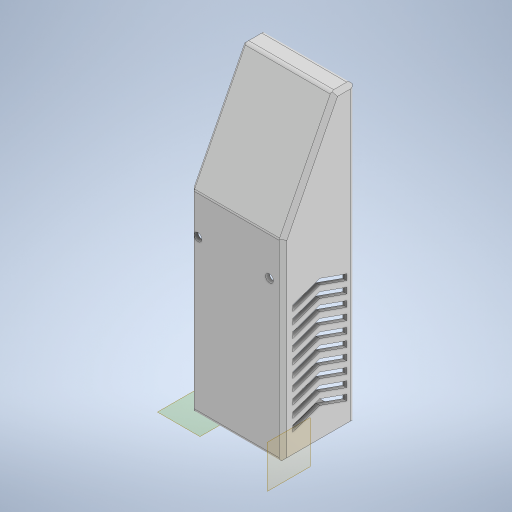
# Autodesk Inventor part: PrawyBłotnik
Saved by Autodesk Inventor 2024 (Build 280153000, 153)
## iProperties
Created: 2025-05-22
Part Number: PrawyBłotnik
Material: Ogólny
Document SubType Name: Modeling
Designer: Victoria
Density: 1 g/cm^3
Appearance: Domyślna
Author: Victoria
Autodesk Inventor part; units mm, degrees
ref_plane "YZ Plane" through (0, 0, 0) normal (1, 0, 0) x (0, 1, 0)
ref_plane "XZ Plane" through (0, 0, 0) normal (0, 1, 0) x (-1, 0, 0)
ref_plane "XY Plane" through (0, 0, 0) normal (0, 0, 1) x (1, 0, 0)
sketch "Szkic1" plane through (0, 0, 0) normal (0, 0, 1) x (1, 0, 0)
  circle A0 centre (16, 0) radius 2
  circle A1 centre (-21, 0) radius 2
  line L0 (-23, 0) -> (-30, 0)
  line L1 (18, 0) -> (23, 0)
  line L2 (23, 0) -> (23, -80)
  line L3 (23, 0) -> (23, 73)
  line L4 (23, 0) -> (96, 0) construction
  line L5 (23, -80) -> (-25, -80)
  line L6 (-25, 73) -> (23, 73)
  line L7 (-25, 73) -> (-25, -80)
  line L8 (-25, 0) -> (-23, 0)
  point P0 (0, 0)
  point P1 (-30, 73)
  point P2 (20.5, 0)
  dimension "d0" = 4
  dimension "d1" = 4
  dimension "d3" = 5
  dimension "d4" = 80
  dimension "d40" = 16
  constraints: 18 end point, 4 horizontal, 2 horizontal alignment, 2 perpendicular, 2 point on line, 1 collinear, 1 midpoint, 1 vertical, 4 other
  measures "d3" distance of L1.start L1.end
  measures "d4" distance of L1.end L2.end
  measures "d40" distance of point (0, 0) point (16, 0)
extrude "Wyciągnięcie proste1" add sketch "Szkic1" along normal blind 2
sketch "Szkic2" plane through (0, 0, 0) normal (0, 0, -1) x (-1, 0, 0)
  line L0 (-23, 73) -> (25, 73) projected
  line L1 (-23, -80) -> (-23, 73) projected
  line L2 (25, -80) -> (-23, -80) projected
  line L3 (25, 73) -> (25, -80) projected
  circle A0 centre (-16, 0) radius 2 projected
  circle A1 centre (21, 0) radius 2 projected
  line L4 (-21, 71) -> (23, 71)
  line L5 (23, 71) -> (23, -78)
  line L6 (23, -78) -> (-21, -78)
  line L7 (-21, -78) -> (-21, 71)
  line L8 (23, 71) -> (25, 71)
  line L9 (23, -78) -> (25, -78)
  line L10 (25, 73) -> (25, -80) projected
  line L11 (23, -68) -> (25, -68)
  line L12 (23, -20) -> (25, -20)
  line L13 (23, 20) -> (25, 20)
  line L14 (23, 10) -> (25, 10)
  point P0 (0, 0)
  dimension "d9" = 2
  constraints: 20 end point, 11 point on line, 5 perpendicular, 3 other
  measures "d9" distance between parallel lines of L1 L7
extrude "Wyciągnięcie proste2" add sketch "Szkic2" along normal blind 35 contours L0 L3 L8 L4 L7 L6 L9 L2 L1 | L3 L13 L5 L8 | L3 L14 L5 L13 | L9 L5 L11 L3
sketch "Szkic3" plane through (23, -80, 2) normal (1, 0, 0) x (0, 0, -1)
  line L0 (37, 153) -> (37, 0) projected
  line L1 (37, 153) -> (27, 153)
  line L2 (0, 0) -> (0, 153) projected
  line L3 (0, 100) -> (27, 153)
  line L4 (0, 100) -> (0, 153)
  line L5 (37, 153) -> (0, 153) projected
  line L6 (27, 153) -> (0, 153)
  point P0 (2, 80)
  dimension "d12" = 10
  dimension "d42" = 20
  constraints: 8 end point, 2 collinear, 1 horizontal, 1 point on line
  measures "d12" distance of L0.start L1.end
  measures "d42" vertical distance of L3.start point (2, 80)
extrude "Wyciągnięcie proste3" cut sketch "Szkic3" against normal up to surface (48 mm away)
sketch "Szkic4" plane through (23, -80, -35) normal (1, 0, 0) x (0, 0, -1)
  line L0 (-37, 100) -> (-10, 153) projected
  line L1 (-37, 100) -> (-35, 100)
  line L2 (-35, 151) -> (-35, 2) projected
  line L3 (0, 153) -> (-10, 153) projected
  line L4 (-10, 153) -> (-8, 153)
  line L5 (-8, 153) -> (-35, 100)
  point P0 (-35, 80)
  point P1 (-35, 103.9259)
  dimension "d15" = 2
  constraints: 6 end point, 2 point on line, 1 horizontal
  measures "d15" distance of L0.end L4.end
extrude "Wyciągnięcie proste4" add sketch "Szkic4" against normal up to surface (48 mm away)
ref_plane "Płaszczyzna konstrukcyjna1" through (23, -77, -1) normal (1, 0, 0) x (0, 0, -1)
sketch "Szkic6" plane through (23, -77, -1) normal (1, 0, 0) x (0, 0, -1)
  line L0 (32, 0) -> (32, 9) projected
  line L1 (32, 9) -> (16, 9)
  line L2 (-1, 9) -> (32, 9) projected
  line L3 (16, 9) -> (16, 95.8634)
  line L4 (16, 9) -> (16, 14)
  line L5 (30, 9) -> (16, 14)
  line L6 (16, 14) -> (2, 9)
  line L7 (30, 9) -> (30, 12)
  line L8 (16, 14) -> (16, 17)
  line L9 (16, 17) -> (30, 12)
  line L10 (2, 9) -> (2, 12)
  line L11 (2, 96.2799) -> (2, 2) projected
  line L12 (2, 12) -> (16, 17)
  line L13 (16, 20) -> (2, 15)
  line L14 (2, 18) -> (16, 23)
  line L15 (2, 15) -> (2, 18)
  line L16 (30, 15) -> (16, 20)
  line L17 (16, 23) -> (30, 18)
  line L18 (30, 15) -> (30, 18)
  line L19 (16, 26) -> (2, 21)
  line L20 (2, 24) -> (16, 29)
  line L21 (2, 21) -> (2, 24)
  line L22 (30, 21) -> (16, 26)
  line L23 (16, 29) -> (30, 24)
  line L24 (30, 21) -> (30, 24)
  line L25 (16, 32) -> (2, 27)
  line L26 (2, 30) -> (16, 35)
  line L27 (2, 27) -> (2, 30)
  line L28 (30, 27) -> (16, 32)
  line L29 (16, 35) -> (30, 30)
  line L30 (30, 27) -> (30, 30)
  line L31 (16, 38) -> (2, 33)
  line L32 (2, 36) -> (16, 41)
  line L33 (2, 33) -> (2, 36)
  line L34 (30, 33) -> (16, 38)
  line L35 (16, 41) -> (30, 36)
  line L36 (30, 33) -> (30, 36)
  line L37 (16, 44) -> (2, 39)
  line L38 (2, 42) -> (16, 47)
  line L39 (2, 39) -> (2, 42)
  line L40 (30, 39) -> (16, 44)
  line L41 (16, 47) -> (30, 42)
  line L42 (30, 39) -> (30, 42)
  line L43 (16, 50) -> (2, 45)
  line L44 (2, 48) -> (16, 53)
  line L45 (2, 45) -> (2, 48)
  line L46 (30, 45) -> (16, 50)
  line L47 (16, 53) -> (30, 48)
  line L48 (30, 45) -> (30, 48)
  line L49 (16, 56) -> (2, 51)
  line L50 (2, 54) -> (16, 59)
  line L51 (2, 51) -> (2, 54)
  line L52 (30, 51) -> (16, 56)
  line L53 (16, 59) -> (30, 54)
  line L54 (30, 51) -> (30, 54)
  line L55 (16, 62) -> (2, 57)
  line L56 (2, 60) -> (16, 65)
  line L57 (2, 57) -> (2, 60)
  line L58 (30, 57) -> (16, 62)
  line L59 (16, 65) -> (30, 60)
  line L60 (30, 57) -> (30, 60)
  line L61 (16, 68) -> (2, 63)
  line L62 (2, 66) -> (16, 71)
  line L63 (2, 63) -> (2, 66)
  line L64 (30, 63) -> (16, 68)
  line L65 (16, 71) -> (30, 66)
  line L66 (30, 63) -> (30, 66)
  point P0 (-1, 77)
  point P1 (0, 9)
  point P2 (16, 71)
  point P3 (2, 63)
  point P4 (16, 65)
  point P5 (2, 57)
  point P6 (16, 59)
  point P7 (2, 54)
  point P8 (2, 51)
  point P9 (16, 53)
  point P10 (2, 48)
  point P11 (2, 45)
  point P12 (2, 39)
  point P13 (2, 33)
  point P14 (2, 27)
  point P15 (16, 29)
  point P16 (2, 21)
  point P17 (16, 23)
  point P18 (2, 18)
  point P19 (2, 15)
  point P20 (16, 17)
  point P21 (2, 148)
  point P22 (2, 104.6118)
  dimension "d22" = 16
  dimension "d23" = 5
  dimension "d24" = 3
  dimension "d25" = 3
  dimension "d26" = 3
  dimension "d29" = 6
  constraints: 128 end point, 6 point on line, 1 perpendicular, 1 vertical, 119 other
  measures "d22" distance of L0.end L1.end
  measures "d23" distance of L1.end L4.end
  measures "d24" distance of L5.start L7.end
  measures "d25" distance of L4.end L8.end
  measures "d26" distance of L6.end L10.end
  measures "d29" distance of L4.end L13.start
extrude "Wyciągnięcie proste5" cut sketch "Szkic6" against normal blind 10 contours L5 L3 L9 L7 | L6 L10 L12 L3 | L13 L11 L14 L3 | L3 L17 L18 L16 | L19 L11 L20 L3 | L3 L23 L24 L22 | L25 L11 L26 L3 | L3 L29 L30 L28 | L31 L11 L32 L3 | L3 L35 L36 L34 | L37 L11 L38 L3 | L3 L41 L42 L40 | L43 L11 L44 L3 | L3 L47 L48 L46 | L49 L11 L50 L3 | L3 L53 L54 L52 | L55 L11 L56 L3 | L3 L59 L60 L58 | L61 L11 L62 L3 | L3 L65 L66 L64
ref_plane "Płaszczyzna konstrukcyjna2" through (-22, -80, 0) normal (0, -1, 0) x (1, 0, 0)
sketch "Szkic7" plane through (-22, -80, 0) normal (0, -1, 0) x (1, 0, 0)
  point P0 (22, 0)
extrude "Wyciągnięcie proste6" [suppressed]
chamfer "Faza2" distance 2 angle 45 16 edges at (23, -80, -16.5) (23, -30, 2) (23, 46.5, -11.5) (23, 73, -30) (21, -29, 0) (21, 45.5, -12.9906) (21, -78, -17.5) (-25, 46.5, -11.5) (-25, 73, -30) (-25, -30, 2) (-25, -80, -16.5) (-23, -78, -17.5) (-23, 15, 0) (-23, 45.5, -12.9906) (-23, 71, -30.4906) (21, 71, -30.4906)
fillet "Zaokrąglenie2" radius 2 8 edges at (-1, -80, 2) (-1, -80, -35) (-1, 20, 2) (-1, 73, -25) (-1, 73, -35) (23, -3.5, -35) (-25, 40.5, -35) (-25, -73.0001, -35)
